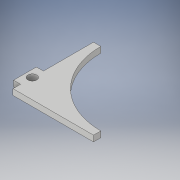
# Autodesk Inventor part: frameClip
Saved by Autodesk Inventor 2019 (Build 230136000, 136)
## iProperties
Created: 2019-09-19
Part Number: frameClip
Material: Generic
Document SubType Name: Modeling
Designer: 19879326
Density: 1 g/cm^3
Appearance: Default
Author: 19879326
Autodesk Inventor part; units mm, degrees
ref_plane "YZ Plane" through (0, 0, 0) normal (1, 0, 0) x (0, 1, 0)
ref_plane "XZ Plane" through (0, 0, 0) normal (0, 1, 0) x (-1, 0, 0)
ref_plane "XY Plane" through (0, 0, 0) normal (0, 0, 1) x (1, 0, 0)
sketch "Sketch1" plane through (0, 0, 0) normal (0, 1, 0) x (-1, 0, 0)
  arc A0 (25, 0) -> (0, 25) centre (0, 0) ccw
  line L0 (27.5, 27.5) -> (0, 27.5)
  line L1 (0, 27.5) -> (0, 25)
  line L2 (27.5, 0) -> (25, 0)
  line L3 (27.5, 24.9) -> (29.9, 24.9)
  line L4 (29.9, 24.9) -> (29.9, 17.1)
  line L5 (29.9, 17.1) -> (27.5, 17.1)
  line L6 (27.5, 27.5) -> (27.5, 24.9)
  line L7 (27.5, 17.1) -> (27.5, 0)
  circle A1 centre (27.5, 20.9) radius 1.5
  point P0 (26.25, 0)
  point P1 (0, 26.25)
  point P2 (27.5, 26.2)
  point P3 (27.5, 8.55)
  dimension "d0" = 50
  dimension "d3" = 2.5
  dimension "d4" = 2.5
  dimension "d5" = 2.4
  dimension "d6" = 2.6
  dimension "d7" = 7.8
  dimension "d8" = 3
  dimension "d9" = 4
  constraints: 16 end point, 6 perpendicular, 4 midpoint, 3 vertical alignment, 2 centre point, 2 point on circle, 1 coincident, 1 horizontal, 1 horizontal alignment, 1 parallel, 1 vertical
  measures "d0" diameter of A0
  measures "d3" distance of L2.start L2.end
  measures "d4" distance of L1.end L0.end
  measures "d5" distance of L3.start L3.end
  measures "d6" distance between parallel lines of L0 L3
  measures "d7" distance of L3.end L4.end
  measures "d8" diameter of A1
  measures "d9" distance from line of L3 A1.centre
extrude "Extrusion1" add sketch "Sketch1" along normal blind 2
body "Solid1"
